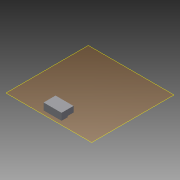
# Autodesk Inventor part: Control_Box
Saved by Autodesk Inventor 2014 SP1 (Build 180222100, 222)
## iProperties
Created: 2015-04-07
Part Number: Control_Box
Material: MDF Medium Density Fiberboard
Document SubType Name: Modeling
Designer: tuleu
Density: 0.8 g/cm^3
Appearance: Cardboard - Corrugated
Author: tuleu
Autodesk Inventor part; units mm, degrees
ref_plane "YZ Plane" through (0, 0, 0) normal (1, 0, 0) x (0, 1, 0)
ref_plane "XZ Plane" through (0, 0, 0) normal (0, 1, 0) x (-1, 0, 0)
ref_plane "XY Plane" through (0, 0, 0) normal (0, 0, 1) x (1, 0, 0)
ref_plane "Work Plane1" through (0, 0, 0) normal (0, 0, 1) x (1, 0, 0)
sketch "Sketch1" plane through (0, 0, 0) normal (0, 0, 1) x (1, 0, 0)
  line L0 (475, -625) -> (475, -525) construction
  line L1 (427.5, -425) -> (532.5, -425) construction
  line L2 (175, -525) -> (175, -625) construction
  line L3 (475, -625) -> (175, -625)
  line L4 (175, -625) -> (175, -425)
  line L5 (175, -425) -> (475, -425)
  line L6 (475, -425) -> (475, -625)
  line L7 (460, -610) -> (190, -610)
  line L8 (190, -610) -> (190, -440)
  line L9 (190, -440) -> (460, -440)
  line L10 (460, -440) -> (460, -610)
  line L11 (325, -625) -> (325, -610) construction
  line L12 (475, -525) -> (460, -525) construction
  line L13 (190, -525) -> (175, -525) construction
  line L14 (325, -440) -> (325, -425) construction
  point P0 (0, 0)
  dimension "d0" = 15
  constraints: 24 end point, 6 midpoint, 5 perpendicular, 4 parallel, 3 equal length, 2 collinear, 2 horizontal
  measures "d0" distance between parallel lines of L3 L7
extrude "Extrusion1" add sketch "Sketch1" along normal blind 100
sketch "Sketch2" plane through (0, 0, 100) normal (0, 0, 1) x (1, 0, 0)
  line L0 (175, -425) -> (475, -425)
  line L1 (475, -425) -> (475, -625)
  line L2 (475, -625) -> (175, -625)
  line L3 (175, -625) -> (175, -425)
  point P0 (0, 0)
  constraints: 8 end point, 2 parallel, 1 horizontal, 1 perpendicular
extrude "Extrusion2" add sketch "Sketch2" along normal blind 15
sketch "Sketch3" plane through (175, -625, 0) normal (-1, 0, 0) x (0, 0, 1)
  line L0 (19, 1250) -> (19, 100) construction
  line L1 (0, 100) -> (-19, 100) construction
  line L2 (0, 200) -> (19, 200)
  line L3 (19, 200) -> (19, 100)
  line L4 (19, 100) -> (0, 100)
  line L5 (0, 100) -> (0, 200)
  point P0 (0, 625)
  constraints: 8 end point, 2 parallel, 1 horizontal, 1 perpendicular
extrude "Extrusion3" cut sketch "Sketch3" against normal up to next
body "Solid1"
